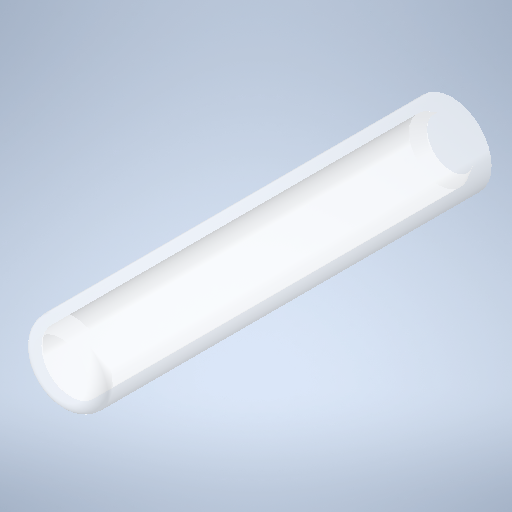
# Autodesk Inventor part: Diffueser
Saved by Autodesk Inventor 2025.3 (Build 293356000, 356)
## iProperties
Created: 2026-01-16
Part Number: Diffueser
Material: Generic
Document SubType Name: Modeling
Designer: Balint
Density: 1 g/cm^3
Appearance: Default
Mass: 26.2568 g
Surface Area: 178.16 cm^2
Volume: 26.2568 cm^3
Author: Balint
Autodesk Inventor part; units mm, degrees
ref_plane "YZ Plane" through (0, 0, 0) normal (1, 0, 0) x (0, 1, 0)
ref_plane "XZ Plane" through (0, 0, 0) normal (0, 1, 0) x (-1, 0, 0)
ref_plane "XY Plane" through (0, 0, 0) normal (0, 0, 1) x (1, 0, 0)
sketch "Sketch4" plane through (0, 0, 0) normal (1, 0, 0) x (0, 1, 0)
  line L0 (-12.5, 0) -> (12.5, 0) projected
  line L1 (-12.5, 0) -> (-9.5, 0)
  line L2 (-9.5, 4.0551) -> (-9.5, 119)
  line L3 (0, 120) -> (0, 123)
  line L4 (0, 123) -> (-8.5, 123)
  arc A0 (-8.5, 123) -> (-12.5, 119) centre (-8.5, 119) ccw
  line L5 (-12.5, 119) -> (-12.5, 0)
  line L6 (-8.5, 120) -> (0, 120)
  arc A1 (-8.5, 120) -> (-9.5, 119) centre (-8.5, 119) ccw
  line L7 (-9.5, 0) -> (-7.9135, 0)
  line L8 (-7.5671, 0.6) -> (-9.4464, 3.8551)
  line L9 (-7.2207, 0) -> (-1.4448, 0) construction
  arc A2 (-9.5, 4.0551) -> (-9.4464, 3.8551) centre (-9.1, 4.0551) ccw
  arc A3 (-7.9135, 0) -> (-7.5671, 0.6) centre (-7.9135, 0.4) ccw
  point P0 (0, 0)
  point P1 (-9.5, 120)
  point P2 (-6.5, 0)
  point P3 (-9.5, 3.9479)
  dimension "d7" = 120
  dimension "d8" = 3
  dimension "d9" = 4
  dimension "d10" = 1
  dimension "d11" = 3
  dimension "d14" = 120
  dimension "d15" = 0.4
  constraints: 18 end point, 9 point on line, 8 point on circle, 7 tangent, 4 centre point, 2 horizontal, 2 perpendicular, 1 equal radius, 1 vertical
  measures "d7" distance of point (-9.5, 120) L1.end
  measures "d8" distance of L3.end L3.start
  measures "d9" radius of A0
  measures "d10" radius of A1
  measures "d11" distance of L1.end point (-6.5, 0)
  measures "d14" angle of L9 L8
  measures "d15" radius of A2
revolve "Revolution1" add sketch "Sketch4" angle 360 about axis through (0, 0, 120) along (0, 0, 1)
body "Solid2"
